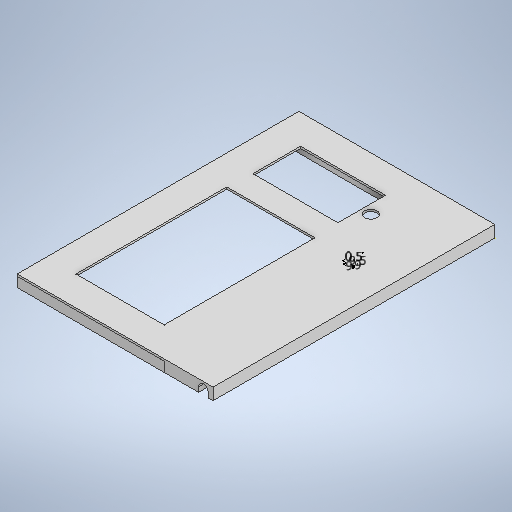
# Autodesk Inventor part: iphone-playbook dock
Saved by Autodesk Inventor 2025 (Build 290162000, 162)
## iProperties
Created: 2024-07-05
Part Number: iphone-playbook dock
Material: Generic
Document SubType Name: Modeling
Designer: colin
Density: 1 g/cm^3
Appearance: Default
Author: colin
Autodesk Inventor part; units mm, degrees
ref_plane "YZ Plane" through (0, 0, 0) normal (1, 0, 0) x (0, 1, 0)
ref_plane "XZ Plane" through (0, 0, 0) normal (0, 1, 0) x (-1, 0, 0)
ref_plane "XY Plane" through (0, 0, 0) normal (0, 0, 1) x (1, 0, 0)
sketch "Sketch1" plane through (0, 0, 0) normal (0, 1, 0) x (-1, 0, 0)
  line L0 (0, 0) -> (0, -194)
  line L1 (0, -194) -> (130, -194)
  line L2 (130, -194) -> (130, 0)
  line L3 (130, 0) -> (0, 0)
  line L4 (0, -194) -> (123.8, -194)
  line L5 (126.866, -194) -> (126.866, -252.6)
  line L6 (126.866, -252.6) -> (3.066, -252.6)
  line L7 (3.066, -252.6) -> (3.066, -194)
  line L8 (140, 0) -> (140, -262.6)
  line L9 (140, -262.6) -> (0, -262.6)
  line L10 (140, 0) -> (140, 10)
  line L11 (-10, 0) -> (-10, -262.6)
  line L12 (-10, -262.6) -> (3.066, -262.6)
  line L13 (140, 10) -> (-10, 10)
  line L14 (-10, 10) -> (-10, 0)
  line L15 (-10, 10) -> (-60, 10)
  line L16 (-60, 10) -> (-60, -262.6)
  line L17 (-60, -262.6) -> (-10, -262.6)
  line L18 (108.366, -194) -> (108.366, -247.6)
  line L19 (21.566, -199) -> (21.566, -247.6)
  line L20 (110, -150.1456) -> (110, -20)
  line L21 (110, -174) -> (20, -174)
  line L22 (110, -174) -> (110, -150.1456)
  line L23 (102.8172, -20) -> (110, -20)
  line L24 (102.8172, -20) -> (20, -20)
  line L25 (20, -41.8625) -> (20, -20)
  line L26 (20, -41.8625) -> (20, -174)
  line L27 (21.566, -199) -> (21.566, -200.5)
  line L28 (108.366, -199) -> (21.566, -199)
  line L29 (108.366, -252.6) -> (108.366, -247.6)
  line L30 (108.366, -247.6) -> (21.566, -247.6)
  line L31 (21.566, -194) -> (12.316, -194)
  line L32 (12.316, -217.05) -> (12.316, -223.3)
  circle A0 centre (12.316, -223.3) radius 6.25
  line L33 (130, -194) -> (130, -252.6)
  line L34 (130, -252.6) -> (126.866, -252.6)
  line L35 (0, -194) -> (0, -252.6)
  line L36 (0, -252.6) -> (3.066, -252.6)
  line L37 (102.8172, -247.6) -> (102.8172, -267.6)
  line L38 (102.8172, -267.6) -> (140, -267.6)
  line L39 (140, -267.6) -> (140, -262.6)
  line L40 (102.8172, -267.6) -> (0, -267.6)
  line L41 (0, -267.6) -> (0, -252.6)
  line L42 (130, -252.6) -> (130, -267.6)
  line L43 (126.866, -252.6) -> (126.866, -267.6)
  line L44 (3.066, -252.6) -> (3.066, -267.6)
  line L45 (3.066, -194) -> (3.066, -217)
  line L46 (3.066, -252.6) -> (3.066, -229.6)
  line L47 (3.066, -217) -> (0, -217)
  line L48 (3.066, -229.6) -> (0, -229.6)
  line L49 (0, -217) -> (-10, -217)
  line L50 (0, -229.6) -> (-10, -229.55)
  line L51 (0, -267.6) -> (-60, -267.6)
  line L52 (-60, -267.6) -> (-60, -262.6)
  line L53 (-10, -262.6) -> (-10, -267.6)
  line L54 (-10, -194) -> (-20, -194)
  line L55 (-20, -194) -> (-20, -174)
  line L56 (-20, -174) -> (-10, -174)
  line L57 (-10, 0) -> (-10, -10)
  line L58 (-10, -10) -> (-20, -10)
  line L59 (-20, -10) -> (-20, 0)
  line L60 (37.3032, -247.6) -> (37.3032, -277.6)
  line L61 (37.3032, -277.6) -> (-60, -277.6)
  line L62 (-60, -277.6) -> (-60, -267.6)
  line L63 (140, -267.6) -> (140, -277.6)
  line L64 (140, -277.6) -> (37.3032, -277.6)
  dimension "d18" = 12.5
  dimension "d0" = 194
  dimension "d1" = 130
  dimension "d2" = 123.8
  dimension "d3" = 58.6
  dimension "d4" = 10
  dimension "d5" = 262.6
  dimension "d6" = 10
  dimension "d7" = 10
  dimension "d8" = 50
  dimension "d14" = 6.5
  dimension "d15" = 5
  dimension "d16" = 5
  dimension "d17" = 9.25
  dimension "d19" = 20
  dimension "d29" = 23
  dimension "d30" = 23
  dimension "d46" = 10
  dimension "d47" = 10
  dimension "d55" = 30
  constraints: 130 end point, 39 perpendicular, 27 point on line, 6 parallel, 3 horizontal, 3 vertical, 1 coincident, 1 vertical alignment, 2 other
  measures "d0" distance of L0.end L0.start
  measures "d1" distance of L1.start L1.end
  measures "d2" distance of L4.start L4.end
  measures "d3" distance of L5.start L5.end
  measures "d4" distance of L2.end L8.start
  measures "d5" distance of L8.start L8.end
  measures "d6" distance of L8.start L10.end
  measures "d7" distance of L0.start L11.start
  measures "d8" distance of L13.end L15.end
  measures "d14" distance of L31.start L27.end
  measures "d15" distance of L18.start L28.start
  measures "d16" distance of L18.end L29.start
  measures "d17" distance of L31.start L31.end
  measures "d19" distance of L37.start L37.end
  measures "d29" distance of L7.end L45.end
  measures "d30" distance of L6.end L46.end
  measures "d46" distance of L54.start L54.end
  measures "d47" distance of L11.start L57.end
  measures "d55" distance of L60.start L60.end
sketch "Sketch2" plane through (0, 0, 0) normal (0, 1, 0) x (-1, 0, 0)
  line L0 (0, 0) -> (0, -194)
  line L1 (0, -194) -> (0, -109)
  line L2 (0, 0) -> (0, -75)
  line L3 (0, -194) -> (0, -119)
  line L4 (0, -119) -> (-10, -119)
  line L5 (-10, -119) -> (-10, -194)
  line L6 (-10, -194) -> (0, -194)
  line L7 (0, -75) -> (-10, -75)
  line L8 (0, 0) -> (-10, 0)
  line L9 (-10, 0) -> (-10, -75)
  line L10 (-10, -262.6) -> (0, -262.6)
  line L11 (0, -262.6) -> (0, -194)
  line L12 (-10, -194) -> (-10, -262.6)
  line L13 (0, -194) -> (0, -262.6)
  line L14 (0, -262.6) -> (3.066, -262.6)
  line L15 (3.066, -262.6) -> (3.066, -252.6)
  line L16 (3.066, -252.6) -> (0, -252.6)
  line L17 (0, -252.6) -> (0, -194)
  line L18 (3.066, -194) -> (3.066, -252.6)
  line L19 (3.066, -252.6) -> (3.066, -224.05)
  line L20 (3.066, -252.6) -> (3.066, -229.6)
  line L21 (3.066, -194) -> (3.066, -217)
  line L22 (3.066, -217) -> (0, -217)
  line L23 (3.066, -229.6) -> (0, -229.6)
  line L24 (0, -217) -> (-10, -217)
  line L25 (0, -229.6) -> (-10, -229.6)
  line L26 (3.066, -252.6) -> (126.866, -252.6)
  line L27 (126.866, -252.6) -> (126.866, -262.6)
  line L28 (126.866, -262.6) -> (3.066, -262.6)
  line L29 (3.066, -252.6) -> (3.066, -262.6)
  line L30 (126.866, -252.6) -> (130, -252.6)
  line L31 (130, -252.6) -> (130, -262.6)
  line L32 (130, -262.6) -> (126.866, -262.6)
  line L33 (130, -252.6) -> (130, 0)
  line L34 (130, 0) -> (0, 0)
  line L35 (130, 0) -> (140, 0)
  line L36 (140, 0) -> (140, -194)
  line L37 (140, -194) -> (140, -252.6)
  line L38 (140, -252.6) -> (130, -252.6)
  line L39 (140, -267.6319) -> (140, -252.6)
  line L40 (140, -267.6319) -> (-10, -267.6319)
  line L41 (-10, -267.6319) -> (-10, -229.6)
  line L42 (-10, 10.006) -> (140, 10.006)
  line L43 (140, 10.006) -> (140, 0)
  line L44 (-10, 10.006) -> (-10, 0)
  line L45 (-10, -75) -> (-10, 0)
  line L46 (0, 0) -> (-10, 0)
  line L47 (0, 0) -> (0, -75)
  line L48 (-10, -75) -> (0, -75)
  line L49 (0, -119) -> (-10, -119)
  line L50 (-10, -194) -> (0, -194)
  line L51 (0, -119) -> (0, -194)
  line L52 (-10, -194) -> (-10, -119)
  line L53 (3.066, -194) -> (0, -194)
  line L54 (3.066, -194) -> (3.066, -217)
  line L55 (-10, -217) -> (3.066, -217)
  line L56 (-10, -217) -> (-10, -194)
  line L57 (-10, -229.6) -> (-10, -267.6319)
  line L58 (3.066, -267.6319) -> (3.066, -229.6)
  line L59 (3.066, -229.6) -> (-9.4866, -229.6)
  line L60 (0, -194) -> (0, 0)
  line L61 (-10, -194) -> (-20, -194)
  line L62 (-20, -194) -> (-20, -184)
  line L63 (-20, -184) -> (-10, -184)
  line L64 (-20, -184) -> (-20, -174)
  line L65 (-20, -174) -> (-10, -174)
  line L66 (-10, -184) -> (-10, -189)
  line L67 (-5, -189) -> (-5, -179)
  line L68 (-5, -179) -> (-15, -179)
  line L69 (-15, -179) -> (-15, -189)
  line L70 (-15, -189) -> (-5, -189)
  line L71 (0, 0) -> (0, 2.5)
  line L72 (0, 2.5) -> (-7.5, 2.5)
  line L73 (-7.5, 2.5) -> (-7.5, 7.5)
  line L74 (-7.5, 7.5) -> (0, 7.5)
  line L75 (0, 7.5) -> (2.5, 7.5)
  line L76 (2.5, 7.5) -> (2.5, 2.5)
  line L77 (2.5, 2.5) -> (0, 2.5)
  line L78 (-10, -282.6) -> (-10, -267.6319)
  line L79 (50.7455, -277.6) -> (-5, -277.6)
  line L80 (-5, -277.6) -> (-5, -257.6)
  line L81 (-5, -257.6) -> (50.7455, -257.6)
  line L82 (50.7455, -257.6) -> (135, -257.6)
  line L83 (135, -257.6) -> (135, -277.6)
  line L84 (135, -277.6) -> (50.7455, -277.6)
  line L85 (140, -277.6) -> (-60, -277.6)
  line L86 (-60, -277.6) -> (-60, -262.6)
  line L87 (-10, -262.6) -> (-60, -262.6)
  line L88 (140, -277.6) -> (140, -267.6319)
  line L89 (3.066, -267.6319) -> (3.066, -272.6159)
  line L90 (3.066, -272.6159) -> (135, -272.6159)
  line L91 (130, -252.6) -> (133, -252.6)
  line L92 (133, -252.6) -> (133, 0)
  line L93 (133, 0) -> (130, 0)
  point P0 (-10, -277.6)
  point P1 (135, -267.6319)
  point P2 (-5, -267.6319)
  point P3 (3.066, -257.6)
  dimension "d22" = 75
  dimension "d23" = 75
  dimension "d24" = 10
  dimension "d25" = 262.6
  dimension "d27" = 23
  dimension "d28" = 23
  dimension "d48" = 10
  dimension "d49" = 10
  dimension "d50" = 10
  dimension "d51" = 2.5
  dimension "d52" = 7.5
  dimension "d53" = 5
  dimension "d54" = 2.5
  dimension "d67" = 3
  constraints: 188 end point, 38 point on line, 34 perpendicular, 18 collinear, 7 vertical, 6 parallel, 4 horizontal
  measures "d22" distance of L0.start L2.end
  measures "d23" distance of L0.end L3.end
  measures "d24" distance of L3.end L4.end
  measures "d25" distance of L8.end L10.start
  measures "d27" distance of L15.end L20.end
  measures "d28" distance of L18.start L21.end
  measures "d48" distance of L5.end L61.end
  measures "d49" distance of L61.end L62.end
  measures "d50" distance of L62.end L64.end
  measures "d51" distance of L0.start L71.end
  measures "d52" distance of L71.end L72.end
  measures "d53" distance of L72.end L73.end
  measures "d54" distance of L74.end L75.end
  measures "d67" distance of L30.end L91.end
extrude "Extrusion1" add sketch "Sketch2" against normal blind 10 contours L0 L7 L9 L8 | L8 L44 L42 L43 L35 L34 | L31 L82 L27 L30 | L38 L39 L40 L83 L82 L31 | L35 L36 L37 L38 L92 | L0 L6 L5 L70 L67 L68 L4 | L27 L82 L81 L15 L26 | L11 L24 L12 L6 | L53 L18 L22 L11 | L15 L81 L11 L16 | L16 L11 L23 L18 | L61 L62 L63 L69 L70 L5 | L5 L68 L69 L63 L64 L65 | L15 L14 L11 L81 | L11 L81 L80 L10 L12 L25 | L40 L88 L85 L83 | L58 L40 L80 L10 L14 | L11 L10 L80 L81 | L89 L90 L83 L84 L79 L80 L40 | L80 L85 L78 L40 | L40 L41 L10 L80 | L41 L78 L85 L86 L87
extrude "Extrusion2" add sketch "Sketch1" along normal blind 2 contours L3 L2 L1 L0 | L0 L35 L49 L11 L14 L13 L10 L8 L9 L42 L33 L2 L3 | L1 L7 L47 L35 | L1 L18 L28 L19 L30 L60 L6 L7 | L47 L7 L48 L35 | L35 L50 L11 L49 | L33 L34 L5 L1 | L48 L7 L36 L35 | L35 L41 L12 L11 L50 | L11 L17 L16 L15 L14 L56 L55 L54 | L5 L6 L29 L18 L1 | L42 L9 L43 L34 | L36 L44 L9 L41 | L54 L55 L56 L11 | L43 L9 L37 L6 | L42 L38 L43 L9 | L9 L39 L38 L42 | L6 L60 L9 L44 | L41 L51 L53 L12 | L9 L44 L40 L41 | L53 L51 L52 L17 | L6 L37 L30 L29 | L43 L38 L37 L9 | L38 L63 L64 L60 L40 | L60 L30 L37 L6 | L6 L37 L9 L60 | L9 L60 L40 L44 | L40 L60 L61 L62 L51 | L37 L40 L60 L9
sketch "Sketch3" plane through (0, 0, 0) normal (0, -1, 0) x (1, 0, 0)
  line L0 (10, -262.6) -> (10, -194) projected
  line L1 (60, -267.6) -> (-140, -267.6) projected
  line L2 (10, -267.6319) -> (60, -267.6)
  line L3 (60, 10) -> (60, -267.6) projected
  line L4 (60, -267.6) -> (60, 10)
  line L5 (10, 10) -> (10, -75) projected
  line L6 (60, 10) -> (10, 10)
  line L7 (10, 10) -> (10, 0)
  line L8 (10, 0) -> (60, 0)
  line L9 (60, 0) -> (50, 0)
  line L10 (50, 0) -> (50.1707, -267.6063)
  line L11 (50.1707, -267.6063) -> (50.1643, -257.6063)
  line L12 (50.1643, -257.6063) -> (10, -257.6319)
  line L13 (50.1643, -257.6063) -> (60, -257.6063)
  point P0 (0, 0)
  point P1 (10, -229.6)
  point P2 (10, -267.6)
  point P3 (50.1707, -267.6)
  dimension "d35" = 10
  dimension "d36" = 10
  constraints: 20 end point, 7 point on line, 5 perpendicular
  measures "d35" distance of L8.end L9.end
  measures "d36" distance of L10.end L11.end
extrude "Extrusion3" add sketch "Sketch3" along normal blind 10
fillet "Fillet2" radius 6.25 4 edges at (10, -5, -75) (10, -5, -119) (10, -5, 0) (50, -5, 0)
fillet "Fillet3" radius 1.25 1 edges at (-3.066, -5, -194)
sketch "Sketch8" plane through (-140, 2, 10) normal (0, 0, 1) x (1, 0, 0)
  line L0 (190.1675, -12) -> (190.1675, -2) projected
  circle A0 centre (190.1675, -7) radius 4.8934
  line L1 (185.2741, -7) -> (185.2741, -11.8934)
  line L2 (185.2741, -11.8934) -> (195.0609, -11.8934)
  line L3 (195.0609, -11.8934) -> (195.0609, -7)
  line L4 (185.2741, -11.8934) -> (185.2741, -12.5715)
  line L5 (185.2741, -12.5715) -> (195.0609, -12.5715)
  line L6 (195.0609, -12.5715) -> (195.0609, -11.8934)
  point P0 (140, -2)
  constraints: 12 end point, 4 perpendicular, 2 point on circle, 2 vertical, 1 centre point, 1 midpoint, 1 tangent
extrude "Extrusion7" cut sketch "Sketch8" against normal blind 299.5
sketch "Sketch9" plane through (0, -10, 0) normal (0, -1, 0) x (1, 0, 0)
  line L0 (-135, -272.6159) -> (-135, -257.6) projected
  line L1 (-135, -272.6159) -> (-135, -257.6)
  line L2 (-135, -257.6) -> (-3.066, -257.6)
  line L3 (-3.066, -257.6) -> (-3.066, -272.6159)
  line L4 (-3.066, -272.6159) -> (-135, -272.6159) projected
  line L5 (-3.066, -272.6159) -> (-135, -272.6159)
  line L6 (5, -189) -> (15, -189) projected
  line L7 (5, -179) -> (5, -189) projected
  line L8 (5, -189) -> (5, -179)
  line L9 (5, -179) -> (15.0244, -179)
  line L10 (15.0244, -179) -> (15.0244, -189)
  line L11 (15.0244, -189) -> (5, -189)
  line L12 (-2.5, 2.5) -> (7.5, 2.5) projected
  line L13 (-2.5, 7.5) -> (-2.5, 2.5) projected
  line L14 (-2.5, 2.5) -> (-2.5, 7.5)
  line L15 (5, -189) -> (5, -188.5)
  line L16 (14.5, -188.5) -> (14.5, -179.5)
  line L17 (14.5, -179.5) -> (5.5, -179.5)
  line L18 (5.5, -179.5) -> (5.5, -188.5)
  line L19 (5.5, -188.5) -> (14.5, -188.5)
  line L20 (60, -277.6) -> (-140, -277.6) projected
  line L21 (-3.566, -271.6357) -> (-3.566, -258.1)
  line L22 (-3.566, -271.6357) -> (-3.566, -272.1159)
  line L23 (-134.5, -271.0768) -> (-134.5, -272.1159)
  line L24 (-134.5, -271.0768) -> (-134.5, -258.1)
  line L25 (-134.5, -272.1159) -> (-3.566, -272.1159)
  line L26 (-3.566, -258.1) -> (-134.5, -258.1)
  line L27 (7.5, 7.5) -> (7.5, 2.5) projected
  line L28 (7.5, 2.5) -> (7.5, 7.5)
  line L29 (-2.5, 2.5) -> (7.5, 2.5)
  line L30 (7.5, 7.5) -> (-2.5, 7.5)
  line L31 (-2.5, 7.5) -> (-2.5, 7)
  line L32 (-2, 7) -> (7, 7)
  line L33 (-2, 3) -> (-2, 7)
  line L34 (7.5, 7.5) -> (7, 7.5)
  line L35 (7, 7) -> (7, 3)
  line L36 (7.5, 2.5) -> (7.5, 3)
  line L37 (7, 3) -> (-2, 3)
  point P0 (0, 0)
  dimension "d68" = 0.5
  dimension "d69" = 9.5
  dimension "d70" = 9
  dimension "d71" = 9
  constraints: 60 end point, 17 perpendicular, 4 equal length, 4 point on line, 2 vertical, 1 horizontal
  measures "d68" distance of L6.start L15.end
  measures "d69" distance of L15.end L16.start
  measures "d70" distance of L16.start L16.end
  measures "d71" distance of L16.end L17.end
body "Solid1"
